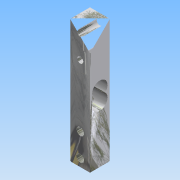
# Autodesk Inventor part: gauge
Saved by Autodesk Inventor 2015 (Build 190159000, 159)
## iProperties
Created: 2015-06-10
Part Number: gauge
Material: Générique
Document SubType Name: Modeling
Designer: Gregwar
Density: 1 g/cm^3
Appearance: Par défaut
Mass: 10.1277 g
Surface Area: 53.5106 cm^2
Volume: 10.1277 cm^3
Author: Gregwar
Autodesk Inventor part; units mm, degrees
ref_plane "YZ Plane" through (0, 0, 0) normal (1, 0, 0) x (0, 1, 0)
ref_plane "XZ Plane" through (0, 0, 0) normal (0, 1, 0) x (-1, 0, 0)
ref_plane "XY Plane" through (0, 0, 0) normal (0, 0, 1) x (1, 0, 0)
sketch "Esquisse1" plane through (0, 0, 0) normal (0, 1, 0) x (-1, 0, 0)
  line L0 (0, 0) -> (12.7, 0)
  line L1 (12.7, 0) -> (12.7, -80)
  line L2 (12.7, -80) -> (0, -80)
  line L3 (0, -80) -> (0, 0)
  line L4 (6.35, 0) -> (6.35, -80) construction
  circle A0 centre (6.35, -5) radius 2
  circle A1 centre (6.35, -20) radius 2
  circle A2 centre (6.35, -75) radius 2.5
  circle A3 centre (6.35, -60) radius 2.5
  line L5 (6.35, -60) -> (6.35, -20) construction
  point P0 (6.35, -40)
  dimension "d0" = 12.7
  dimension "d1" = 80
  dimension "d2" = 40
  dimension "d3" = 15
  dimension "d4" = 15
  dimension "d5" = 4
  dimension "d6" = 5
  constraints: 12 end point, 4 centre point, 4 midpoint, 4 point on line, 2 equal radius, 2 parallel, 1 collinear, 1 horizontal, 1 perpendicular
  measures "d0" distance of L0.start L0.end
  measures "d1" distance of L2.end L0.start
  measures "d2" distance of L5.end L5.start
  measures "d3" distance of A0.centre L5.end
  measures "d4" distance of L5.start A2.centre
  measures "d5" diameter of A0
  measures "d6" diameter of A3
extrude "Extrusion1" add sketch "Esquisse1" along normal blind 12.7
sketch "Esquisse2" plane through (0, 0, 0) normal (1, 0, 0) x (0, 0, -1)
  line L0 (80, 0) -> (0, 0) construction
  line L1 (80, 0) -> (80, 12.7) construction
  line L2 (0, 12.7) -> (80, 12.7) construction
  line L3 (0, 0) -> (0, 12.7) construction
  line L4 (0, 12.7) -> (80, 12.7) construction
  line L5 (40, 12.7) -> (40, 0) construction
  circle A0 centre (43.5, 6.35) radius 5
  line L6 (43.5, 6.35) -> (36.5, 6.35) construction
  circle A1 centre (36.5, 6.35) radius 5
  point P0 (40, 6.35)
  dimension "d9" = 7
  dimension "d10" = 10
  constraints: 4 end point, 4 midpoint, 2 centre point, 1 coincident, 1 equal radius, 1 perpendicular
  measures "d9" distance of A1.centre L6.start
  measures "d10" diameter of A0
extrude "Extrusion2" cut sketch "Esquisse2" against normal through all
